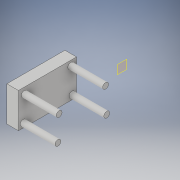
# Autodesk Inventor part: Table
Saved by Autodesk Inventor 2019 (Build 230136000, 136)
## iProperties
Created: 2018-12-11
Part Number: Table
Material: Generic
Document SubType Name: Modeling
Designer: User
Density: 1 g/cm^3
Appearance: Default
Author: User
Autodesk Inventor part; units mm, degrees
ref_plane "XZ Plane" through (0, 0, 0) normal (0, 1, 0) x (-1, 0, 0)
ref_plane "XY Plane" through (0, 0, 0) normal (0, 0, 1) x (1, 0, 0)
ref_plane "Work Plane1" through (3.175, 0, 0) normal (1, 0, 0) x (0, 1, 0)
sketch "Sketch1" plane through (3.175, 0, 0) normal (1, 0, 0) x (0, 1, 0)
  line L0 (93.6959, 280.1689) -> (17.4959, 280.1689)
  line L1 (17.4959, 280.1689) -> (17.4959, 153.1689)
  line L2 (17.4959, 153.1689) -> (93.6959, 153.1689)
  line L3 (93.6959, 153.1689) -> (93.6959, 280.1689)
  point P0 (0, 0)
  dimension "d1" = 127
  dimension "d2" = 76.2
  constraints: 8 end point, 2 parallel, 1 horizontal, 1 perpendicular
  measures "d1" distance of L0.end L1.end
  measures "d2" distance between parallel lines of L1 L3
extrude "Extrusion1" add sketch "Sketch1" along normal blind 25.4
sketch "Sketch2" plane through (28.575, 0, 0) normal (1, 0, 0) x (0, 0, -1)
  circle A0 centre (-270.0089, 27.6559) radius 6.35
  line L0 (-280.1689, 93.6959) -> (-280.1689, 17.4959) projected
  line L1 (-280.1689, 17.4959) -> (-153.1689, 17.4959) projected
  line L2 (-153.1689, 17.4959) -> (-153.1689, 93.6959) projected
  line L3 (-153.1689, 93.6959) -> (-280.1689, 93.6959) projected
  circle A1 centre (-165.8689, 83.5359) radius 6.35
  circle A2 centre (-165.8689, 83.5359) radius 6.35
  circle A3 centre (-165.8689, 83.5359) radius 6.35
  line L4 (-153.1689, 17.4959) -> (-153.1689, 93.6959) projected
  circle A4 centre (-267.4689, 80.9959) radius 6.35
  circle A5 centre (-163.3289, 27.6559) radius 6.35
  point P0 (0, 0)
  dimension "d5" = 12.7
  dimension "d6" = 10.16
  dimension "d7" = 10.16
  dimension "d8" = 10.16
  dimension "d9" = 12.7
  dimension "d10" = 12.7
  dimension "d11" = 12.7
  dimension "d12" = 12.7
  dimension "d13" = 12.7
  dimension "d14" = 12.7
  dimension "d15" = 10.16
  dimension "d16" = 10.16
  constraints: 6 centre point, 2 coincident, 2 concentric
  measures "d5" diameter of A0
  measures "d6" distance from line of A0.centre L0
  measures "d7" distance from line of L1 A0.centre
  measures "d8" distance from line of L3 A3.centre
  measures "d9" distance from line of L4 A3.centre
  measures "d10" diameter of A1
  measures "d11" diameter of A4
  measures "d12" distance from line of L0 A4.centre
  measures "d13" distance from line of A4.centre L3
  measures "d14" diameter of A5
  measures "d15" distance from line of L2 A5.centre
  measures "d16" distance from line of L1 A5.centre
extrude "Extrusion2" add sketch "Sketch2" along normal blind 76.2 contours A0 | A1 | A4 | A5
equation "\"d7\" = d6"
equation "\"d8\" = d7"
equation "\"d9\" = d5"
equation "\"d10\" = d5"
equation "\"d11\" = d5"
equation "\"d12\" = d9"
equation "\"d13\" = d12"
equation "\"d14\" = d5"
equation "\"d15\" = d6"
equation "\"d16\" = d6"
body "Solid1"
